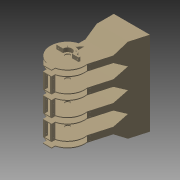
# Autodesk Inventor part: 装填斗
Saved by Autodesk Inventor 2015 (Build 190159000, 159)
## iProperties
Created: 2017-05-03
Part Number: 装填斗
Material: 常规
Document SubType Name: Modeling
Designer: Administrator
Density: 1 g/cm^3
Appearance: 麦色
Author: Administrator
Autodesk Inventor part; units mm, degrees
ref_plane "YZ Plane" through (0, 0, 0) normal (1, 0, 0) x (0, 1, 0)
ref_plane "XZ Plane" through (0, 0, 0) normal (0, 1, 0) x (-1, 0, 0)
ref_plane "XY Plane" through (0, 0, 0) normal (0, 0, 1) x (1, 0, 0)
sketch "草图1" plane through (0, 0, 0) normal (0, 0, 1) x (1, 0, 0)
  circle A0 centre (0, 0) radius 100
  line L0 (-30, 95.3939) -> (-30, 300)
  line L1 (-30, 300) -> (180.1981, 300)
  line L2 (180.1981, 300) -> (98.9752, 14.2797)
  line L3 (96.8246, 25) -> (175, 300)
  dimension "d0" = 200
  dimension "d2" = 30
  dimension "d3" = 300
  dimension "d5" = 205
  dimension "d6" = 25
  dimension "d7" = 5
  constraints: 8 end point, 3 point on circle, 1 centre point, 1 coincident, 1 parallel, 1 perpendicular, 1 point on line, 1 vertical
  measures "d0" diameter of A0
  measures "d2" distance from line of point (0, 0) L0
  measures "d3" distance from line of point (0, 0) L1
  measures "d5" distance of L0.end L3.end
  measures "d6" vertical distance of point (0, 0) L3.start
  measures "d7" distance between parallel lines of L3 L2
extrude "拉伸1" add sketch "草图1" against normal blind 490 contours A0 L3 L1 L2 | L0 L1 L3 A0
sketch "草图3" plane through (-30, 95.3939, 0) normal (-1, 0, 0) x (0, 0, 1)
  line L0 (-490, 204.6061) -> (-490, -81.1142) projected
  line L1 (0, -81.1142) -> (0, 204.6061) projected
  line L2 (-444, 38.8858) -> (-444, -81.1142)
  line L3 (0, 0) -> (-490, 0) projected
  line L4 (-406, 38.8858) -> (-406, -81.1142)
  line L5 (-324, 38.8858) -> (-324, -81.1142)
  line L6 (0, -81.1142) -> (-490, -81.1142) projected
  line L7 (-286, 38.8858) -> (-286, -81.1142)
  line L8 (-166, 38.8858) -> (-166, -81.1142)
  line L9 (-204, 38.8858) -> (-204, -81.1142)
  line L10 (-84, 38.8858) -> (-84, -81.1142)
  line L11 (-46, 38.8858) -> (-46, -81.1142)
  line L12 (-444, 38.8858) -> (-490, 105.1077)
  line L13 (-490, 105.1077) -> (0, 105.1077)
  line L14 (-406, 38.8858) -> (-365, 105.1077)
  line L15 (-324, 38.8858) -> (-365, 105.1077)
  line L16 (-286, 38.8858) -> (-245, 105.1077)
  line L17 (-204, 38.8858) -> (-245, 105.1077)
  line L18 (-166, 38.8858) -> (-125, 105.1077)
  line L19 (-84, 38.8858) -> (-125, 105.1077)
  line L20 (-46, 38.8858) -> (0, 105.1077)
  line L21 (0, 204.6061) -> (-490, 204.6061) projected
  line L22 (-388.0639, 77.354) -> (-365, 114.6061)
  line L23 (-365, 114.6061) -> (-341.0065, 75.8526)
  line L24 (-490, 105.1077) -> (-490, -81.1142)
  line L25 (0, -81.1142) -> (-490, -81.1142)
  line L26 (0, -81.1142) -> (0, 105.1077)
  point P0 (0, -95.3939)
  dimension "d15" = 46
  dimension "d16" = 38
  dimension "d17" = 82
  dimension "d18" = 38
  dimension "d19" = 82
  dimension "d20" = 38
  dimension "d21" = 82
  dimension "d22" = 38
  dimension "d23" = 46
  dimension "d25" = 120
  dimension "d26" = 5
  dimension "d27" = 5
  dimension "d28" = 90
  constraints: 44 end point, 9 equal length, 7 parallel, 4 point on line, 3 perpendicular, 2 collinear, 2 vertical, 1 midpoint, 9 other
  measures "d15" distance between parallel lines of L0 L2
  measures "d16" distance between parallel lines of L2 L4
  measures "d17" distance between parallel lines of L5 L4
  measures "d18" distance between parallel lines of L7 L5
  measures "d19" distance between parallel lines of L9 L7
  measures "d20" distance between parallel lines of L8 L9
  measures "d21" distance between parallel lines of L10 L8
  measures "d22" distance between parallel lines of L11 L10
  measures "d23" distance between parallel lines of L1 L11
  measures "d25" distance of L2.start L2.end
  measures "d26" distance between parallel lines of L14 L22
  measures "d27" distance between parallel lines of L15 L23
  measures "d28" distance from line of L21 L22.end
extrude "拉伸2" cut sketch "草图3" against normal blind 200 contours L12 L2 L3 L0 | L3 L2 L6 L0 | L1 L3 L11 L20 | L15 L5 L3 L4 L14 | L1 L6 L11 L3 | L19 L10 L3 L8 L18 | L3 L5 L6 L4 | L17 L9 L3 L7 L16 | L10 L6 L8 L3 | L3 L9 L6 L7
shell "抽壳1" thickness 5 removed faces 5 at (110.1321, 300, -163.3333) at (39.4896, 91.8726, -311.3333) at (39.4896, 91.8726, -191.3333) at (43.5298, 90.0286, -71.3333) at (39.4896, 91.8726, -431.3333)
sketch "草图4" plane through (-30, 95.3939, -46) normal (0, 0, 1) x (1, 0, 0)
  circle A0 centre (30, -95.3939) radius 100
  arc A1 (128.9752, -81.1142) -> (0, 0) centre (30, -95.3939) ccw projected
  constraints: 1 centre point, 1 coincident, 1 concentric
extrude "拉伸3" add sketch "草图4" against normal blind 5
pattern_linear "矩形阵列1" count 2 spacing 33 along (0, 0, -1) of "拉伸3"
pattern_linear "矩形阵列2" count 4 spacing 120 along (0, 0, -1) of "拉伸3", "矩形阵列1"
sketch "草图5" plane through (-30, 134.2797, -46) normal (0, 0, 1) x (1, 0, 0)
  circle A0 centre (30, -134.2797) radius 15
  dimension "d40" = 30
  constraints: 1 centre point, 1 coincident
  measures "d40" diameter of A0
extrude "拉伸4" cut sketch "草图5" against normal up to surface (398 mm away)
sketch "草图6" plane through (-30, 134.2797, -46) normal (0, 0, 1) x (1, 0, 0)
  line L0 (26, -117.6229) -> (34, -117.6229)
  line L1 (34, -117.6229) -> (34, -119.8229)
  line L2 (34, -119.8229) -> (26, -119.8229)
  line L3 (26, -119.8229) -> (26, -117.6229)
  circle A0 centre (30, -134.2797) radius 15 projected
  dimension "d43" = 8
  dimension "d44" = 2.2
  constraints: 8 end point, 2 parallel, 2 point on circle, 1 horizontal, 1 perpendicular
  measures "d43" distance of L0.start L0.end
  measures "d44" distance of L0.end L1.end
extrude "拉伸5" cut sketch "草图6" against normal blind 5 contours L0 L1 A0 L3
pattern_linear "矩形阵列3" count 4 spacing 120 along (0, 0, -1) of "拉伸5"
sketch "草图7" plane through (-30, 134.2797, -46) normal (0, 0, 1) x (1, 0, 0)
  line L0 (5, -231.1043) -> (55, -231.1043)
  line L1 (55, -231.1043) -> (55, -252.2797)
  line L2 (55, -252.2797) -> (5, -252.2797)
  line L3 (5, -252.2797) -> (5, -231.1043)
  arc A0 (0, -38.8858) -> (128.9752, -120) centre (30, -134.2797) ccw projected
  line L4 (30, -234.2797) -> (30, -252.2797)
  dimension "d50" = 50
  dimension "d51" = 18
  constraints: 10 end point, 3 point on circle, 2 parallel, 1 horizontal, 1 midpoint, 1 perpendicular, 1 point on line
  measures "d50" distance of L1.end L2.end
  measures "d51" distance of L4.start L4.end
extrude "拉伸6" add sketch "草图7" against normal up to surface (398 mm away) contours A0 L4 L2 L3 | L1 L2 L4 A0
sketch "草图8" plane through (-25, -118, -46) normal (0, -1, 0) x (1, 0, 0)
  line L0 (0, -33) -> (50, -33)
  line L1 (50, -33) -> (50, -5)
  line L2 (50, -5) -> (0, -5)
  line L3 (0, -5) -> (0, -33)
  line L4 (0, 0) -> (0, -398) projected
  line L5 (50, 0) -> (50, -398) projected
  line L6 (0, -33) -> (153.2944, -33) projected
  line L7 (0, -5) -> (153.3352, -5) projected
  point P0 (25, 46)
  constraints: 8 end point, 4 collinear, 2 parallel, 1 horizontal, 1 perpendicular
extrude "拉伸7" cut sketch "草图8" against normal up to surface
pattern_linear "矩形阵列4" count 4 spacing 120 along (0, 0, -1) of "拉伸7"
sketch "草图9" plane through (-25, -118, -171) normal (0, -1, 0) x (1, 0, 0)
  line L0 (10, 5) -> (40, 5)
  line L1 (40, 5) -> (40, 87)
  line L2 (40, 87) -> (10, 87)
  line L3 (10, 87) -> (10, 5)
  line L4 (-5, 5) -> (158.0881, 5) projected
  line L5 (-5, 87) -> (158.0881, 87) projected
  line L6 (0, 87) -> (0, 5) projected
  line L7 (50, 92) -> (50, 0) projected
  point P0 (25, 171)
  dimension "d59" = 10
  dimension "d60" = 10
  constraints: 8 end point, 2 collinear, 2 parallel, 1 horizontal, 1 perpendicular
  measures "d59" distance between parallel lines of L6 L3
  measures "d60" distance between parallel lines of L7 L1
extrude "拉伸8" cut sketch "草图9" against normal up to surface contours L3 L2 L1 L0
pattern_linear "矩形阵列5" count 3 spacing 120 along (0, 0, -1) of "拉伸8"
sketch "草图10" plane through (-25, -118, -171) normal (-1, 0, 0) x (0, 0, 1)
  circle A0 centre (72, 10) radius 2.5
  circle A1 centre (20, 10) radius 2.5
  line L0 (92, 0) -> (0, 0) projected
  line L1 (0, 21.1754) -> (0, 0) projected
  line L2 (92, 0) -> (92, 21.1754) projected
  point P0 (171, 118)
  dimension "d66" = 5
  dimension "d67" = 5
  dimension "d68" = 10
  dimension "d69" = 10
  dimension "d70" = 20
  dimension "d71" = 20
  constraints: 2 centre point
  measures "d66" diameter of A0
  measures "d67" diameter of A1
  measures "d68" distance from line of L0 A0.centre
  measures "d69" distance from line of L0 A1.centre
  measures "d70" distance from line of L1 A1.centre
  measures "d71" distance from line of L2 A0.centre
extrude "拉伸9" cut sketch "草图10" against normal up to surface (50 mm away)
thread "螺纹5" size "M5x0.8" class "6H" standard "ANSI Metric M Profile" full length
thread "螺纹6" size "M5x0.8" class "6H" standard "ANSI Metric M Profile" full length
thread "螺纹7" size "M5x0.8" class "6H" standard "ANSI Metric M Profile" full length
thread "螺纹8" size "M5x0.8" class "6H" standard "ANSI Metric M Profile" full length
pattern_linear "矩形阵列7" count 3 spacing 120 along (0, 0, -1) of "拉伸9"
sketch "草图11" plane through (-30, 300, -490) normal (-1, 0, 0) x (0, 0, 1)
  circle A0 centre (436, -187.43) radius 2.5
  circle A1 centre (414, -187.43) radius 2.5
  line L0 (444, -204.6061) -> (444, -165.7203) projected
  line L1 (406, -165.7203) -> (406, -204.6061) projected
  line L2 (444, -418) -> (439, -418) projected
  point P0 (490, -300)
  dimension "d96" = 5
  dimension "d97" = 5
  dimension "d98" = 8
  dimension "d99" = 8
  dimension "d100" = 230.57
  dimension "d101" = 230.57
  constraints: 2 centre point
  measures "d96" diameter of A0
  measures "d97" diameter of A1
  measures "d98" distance from line of L0 A0.centre
  measures "d99" distance from line of L1 A1.centre
  measures "d100" distance from line of L2 A0.centre
  measures "d101" distance from line of L2 A1.centre
extrude "拉伸10" cut sketch "草图11" against normal blind 5
thread "螺纹9" size "M5x0.8" class "6H" standard "ANSI Metric M Profile" full length
thread "螺纹10" size "M5x0.8" class "6H" standard "ANSI Metric M Profile" full length
pattern_linear "矩形阵列8" count 4 spacing 120 along (0, 0, -1) of "拉伸10"
sketch "草图12" plane through (180.1981, 300, 0) normal (0.961889, -0.2734403, 0) x (0, 0, -1)
  circle A0 centre (414, -282.0408) radius 2.5
  circle A1 centre (436, -282.0408) radius 2.5
  line L0 (444, -297.0408) -> (444, -172.2863) projected
  line L1 (406, -172.2863) -> (406, -297.0408) projected
  line L2 (411, -297.0408) -> (439, -297.0408) projected
  point P0 (0, -337.8401)
  dimension "d111" = 5
  dimension "d112" = 5
  dimension "d113" = 8
  dimension "d114" = 8
  dimension "d115" = 15
  dimension "d116" = 15
  constraints: 2 centre point
  measures "d111" diameter of A0
  measures "d112" diameter of A1
  measures "d113" distance from line of L0 A1.centre
  measures "d114" distance from line of L1 A0.centre
  measures "d115" distance from line of L2 A1.centre
  measures "d116" distance from line of L2 A0.centre
extrude "拉伸11" cut sketch "草图12" against normal blind 5
thread "螺纹11" size "M5x0.8" class "6H" standard "ANSI Metric M Profile" full length
thread "螺纹12" size "M5x0.8" class "6H" standard "ANSI Metric M Profile" full length
pattern_linear "矩形阵列9" count 4 spacing 120 along (0, 0, 1) of "拉伸11"
sketch "草图13" plane through (-30, 134.2797, -46) normal (0, 0, 1) x (1, 0, 0)
  line L0 (95, -124.2797) -> (95, -134.2797)
  line L1 (-35, -134.2797) -> (-35, -124.2797)
  arc A0 (73.8748, -124.2797) -> (-13.8748, -124.2797) centre (30, -134.2797) ccw
  arc A1 (56, -134.2797) -> (4, -134.2797) centre (30, -134.2797) ccw
  line L2 (95, -134.2797) -> (56, -134.2797)
  line L3 (4, -134.2797) -> (-35, -134.2797)
  line L4 (-35, -124.2797) -> (6, -124.2797)
  line L5 (54, -124.2797) -> (95, -124.2797)
  circle A2 centre (30, -134.2797) radius 15 projected
  line L6 (30, -134.2797) -> (30, -142.9323)
  dimension "d126" = 45
  dimension "d127" = 26
  dimension "d128" = 10
  dimension "d129" = 10
  dimension "d130" = 8.6526
  dimension "d131" = 130
  constraints: 14 end point, 6 point on circle, 5 parallel, 4 point on line, 2 centre point, 2 concentric, 2 horizontal, 2 perpendicular, 1 vertical, 1 other
  measures "d126" radius of A0
  measures "d127" radius of A1
  measures "d128" distance of L0.start L0.end
  measures "d129" distance of L1.start L1.end
  measures "d130" distance of L6.start L6.end
  measures "d131" distance between parallel lines of L0 L1
extrude "拉伸12" add sketch "草图13" along normal blind 23 contours L0 L2 A1 L5 | L5 A1 L4 A0 | L4 A1 L3 L1
sketch "草图14" plane through (-65, 10, -46) normal (0, 1, 0) x (1, 0, 0)
  circle A0 centre (10, -11.5) radius 4
  line L0 (0, 0) -> (0, -23) projected
  line L1 (21.1252, -23) -> (0, -23) projected
  circle A1 centre (120, -11.5) radius 4
  line L2 (108.8748, 0) -> (130, 0) projected
  point P0 (65, -46)
  dimension "d134" = 8
  dimension "d135" = 10
  dimension "d136" = 11.5
  dimension "d137" = 8
  dimension "d138" = 110
  dimension "d139" = 11.5
  constraints: 2 centre point
  measures "d134" diameter of A0
  measures "d135" distance from line of L0 A0.centre
  measures "d136" distance from line of L1 A0.centre
  measures "d137" diameter of A1
  measures "d138" distance of A1.centre A0.centre
  measures "d139" distance from line of L2 A1.centre
extrude "拉伸13" cut sketch "草图14" against normal through all
sketch "草图15" plane through (-30, 134.2797, -23) normal (0, 0, 1) x (1, 0, 0)
  line L0 (27, -39.3798) -> (33, -39.3798)
  line L1 (33, -39.3798) -> (33, -89.3798)
  line L2 (33, -89.3798) -> (27, -89.3798)
  line L3 (27, -89.3798) -> (27, -39.3798)
  arc A0 (33, -89.3798) -> (27, -89.3798) centre (30, -134.2797) ccw
  arc A1 (73.8748, -124.2797) -> (-13.8748, -124.2797) centre (30, -134.2797) ccw projected
  dimension "d142" = 6
  dimension "d143" = 50
  constraints: 8 end point, 2 concentric, 2 parallel, 2 point on circle, 1 centre point, 1 horizontal, 1 perpendicular
  measures "d142" distance of L0.start L0.end
  measures "d143" distance of L0.end L1.end
extrude "拉伸14" add sketch "草图15" against normal blind 23 contours L0 L1 A0 L3
pattern_linear "矩形阵列10" count 2 spacing 421 along (0, 0, -1) of "拉伸12", "拉伸13", "拉伸14"
chamfer "倒角1" distance 50 distance2 23 1 edges at (0, 94.8999, -23) measured on face at (44.9583, 3.3333, -23)
chamfer "倒角2" distance 50 distance2 23 1 edges at (0, 94.8999, -467) measured on face at (44.9583, 3.3333, -467)
sketch "草图16" plane through (-30, 134.2797, -23) normal (0, 0, 1) x (1, 0, 0)
  circle A0 centre (4.8977, -109.1774) radius 2.5
  circle A1 centre (55.1023, -109.1774) radius 2.5
  arc A2 (55.1023, -109.1774) -> (4.8977, -109.1774) centre (30, -134.2797) ccw
  circle A3 centre (30, -134.2797) radius 15 projected
  line L0 (55.1023, -109.1774) -> (30, -134.2797)
  line L1 (30, -134.2797) -> (4.8977, -109.1774)
  line L2 (30, -134.2797) -> (43.1413, -134.2797)
  dimension "d155" = 5
  dimension "d156" = 5
  dimension "d157" = 35.5
  dimension "d158" = 13.1413
  dimension "d159" = 45
  constraints: 6 end point, 3 centre point, 2 point on circle, 1 concentric, 1 horizontal, 1 perpendicular
  measures "d155" diameter of A0
  measures "d156" diameter of A1
  measures "d157" radius of A2
  measures "d158" distance of L0.end L2.end
  measures "d159" angle of L2 L0
extrude "拉伸15" cut sketch "草图16" against normal blind 23 contours A0 L1 A2 | A2 L1 A0 | A2 L0 A1 | A1 L0 A2
thread "螺纹13" size "M5x0.8" class "6H" standard "ANSI Metric M Profile" full length
thread "螺纹14" size "M5x0.8" class "6H" standard "ANSI Metric M Profile" full length
sketch "草图17" plane through (0, 0, -467) normal (0, 0, -1) x (-1, 0, 0)
  circle A0 centre (-25.1023, 25.1023) radius 2.5
  circle A1 centre (25.1023, 25.1023) radius 2.5
  circle A2 centre (-25.1023, 25.1023) radius 2.5 projected
  circle A3 centre (25.1023, 25.1023) radius 2.5 projected
  arc A4 (25.1023, 25.1023) -> (-25.1023, 25.1023) centre (0, 0) ccw
  arc A5 (26, 0) -> (-26, 0) centre (0, 0) ccw projected
  point P0 (0, 0)
  dimension "d166" = 5
  dimension "d167" = 5
  dimension "d174" = 35.5
  constraints: 3 centre point, 3 concentric, 2 point on circle
  measures "d166" diameter of A0
  measures "d167" diameter of A1
  measures "d174" radius of A4
extrude "拉伸16" cut sketch "草图17" against normal blind 23
thread "螺纹15" size "M5x0.8" class "6H" standard "ANSI Metric M Profile" full length
thread "螺纹16" size "M5x0.8" class "6H" standard "ANSI Metric M Profile" full length
